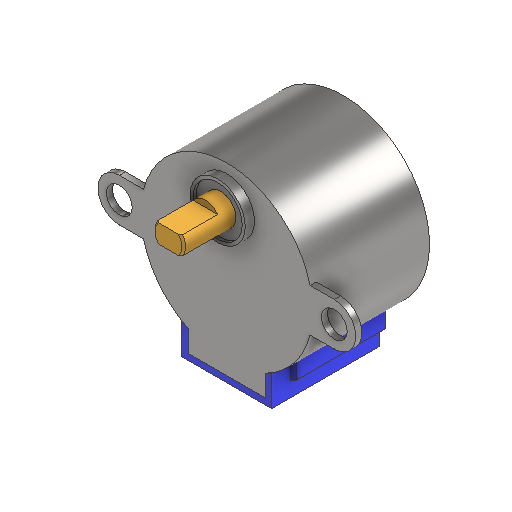
# Autodesk Inventor part: 28BYJ-48 Stepper
Saved by Autodesk Inventor 2023 (Build 270158000, 158)
## iProperties
Created: 2019-05-19
Part Number: 28BYJ-48 Stepper
Material: Generic
Document SubType Name: Modeling
Designer: jotap
Density: 1 g/cm^3
Appearance: Semi-Polished
Author: jotap
Autodesk Inventor part; units mm, degrees
ref_plane "YZ Plane" through (0, 0, 0) normal (1, 0, 0) x (0, 1, 0)
ref_plane "XZ Plane" through (0, 0, 0) normal (0, 1, 0) x (-1, 0, 0)
sketch "Sketch1" plane through (0, 0, 0) normal (0, 0, 1) x (1, 0, 0)
  line L0 (0, 19.6) -> (0, -19.6) construction
  line L1 (-19.6, 0) -> (19.6, 0) construction
  circle A0 centre (0, 0) radius 14
  dimension "d0" = 28
  constraints: 1 centre point, 1 coincident
  measures "d0" diameter of A0
extrude "Extrusion1" add sketch "Sketch1" against normal blind 19
sketch "Sketch2" plane through (0, 0, 0) normal (0, 0, 1) x (1, 0, 0)
  circle A0 centre (0, 0) radius 14 construction
  circle A1 centre (0, 8) radius 4.5
  dimension "d3" = 9
  dimension "d4" = 8
  constraints: 1 centre point
  measures "d3" diameter of A1
  measures "d4" distance of A1.centre A0.centre
extrude "Extrusion2" add sketch "Sketch2" along normal blind 1.5
sketch "Sketch3" plane through (0, 8, 1.5) normal (0, 0, 1) x (1, 0, 0)
  circle A0 centre (0, 0) radius 4.5 construction
  circle A1 centre (0, 0) radius 2.5
  point P0 (0, -8)
  dimension "d7" = 5
  constraints: 1 centre point, 1 coincident
  measures "d7" diameter of A1
extrude "Extrusion3" add sketch "Sketch3" along normal blind 2
sketch "Sketch4" plane through (0, 8, 3.5) normal (0, 0, 1) x (1, 0, 0)
  circle A0 centre (0, 0) radius 2.5 construction
  line L0 (-1.9908, 1.5122) -> (2.0091, 1.4878)
  line L1 (0, 11.6) -> (0, -27.6) construction
  line L2 (-2.6789, 0.0164) -> (3.364, -0.0205) construction
  line L3 (-2.0091, -1.4878) -> (1.9908, -1.5122)
  arc A1 (-1.9908, 1.5122) -> (-2.0091, -1.4878) centre (0, 0) ccw
  arc A2 (1.9908, -1.5122) -> (2.0091, 1.4878) centre (0, 0) ccw
  point P0 (0, -8)
  dimension "d10" = 1.5
  constraints: 6 end point, 4 point on circle, 2 centre point, 2 symmetric about line
  measures "d10" distance from line of L0 A0.centre
extrude "Extrusion4" add sketch "Sketch4" along normal blind 6
chamfer "Chamfer1" distance 0.3 angle 45 2 edges at (2.5, 7.9847, 9.5) (-2.5, 8.0153, 9.5)
sketch "Sketch5" plane through (0, 8, 1.5) normal (0, 0, 1) x (1, 0, 0)
  circle A0 centre (0, 0) radius 4.5 construction
  line L0 (-12.0062, 0) -> (13.0923, 0) construction
  line L1 (0, 11.6) -> (0, -27.6) construction
  circle A1 centre (0, 0) radius 4
  circle A2 centre (0, 0) radius 2.5
  point P0 (0, -8)
  dimension "d16" = 8
  constraints: 2 centre point, 2 coincident, 2 end point, 1 horizontal
  measures "d16" diameter of A1
extrude "Extrusion5" cut sketch "Sketch5" against normal blind 0.5
sketch "Sketch6" plane through (0, 0, 0) normal (0, 0, 1) x (1, 0, 0)
  circle A0 centre (0, 0) radius 14 construction
  arc A1 (-17.5, 3.5) -> (-17.5, -3.5) centre (-17.5, 0) ccw
  line L0 (0, 19.6) -> (0, -19.6) construction
  line L1 (-31.0119, 0) -> (21.502, 0) construction
  circle A2 centre (-17.5, 0) radius 2.1
  line L2 (-17.5, 3.5) -> (-13.5554, 3.5)
  line L3 (-17.5, -3.5) -> (-13.5554, -3.5)
  arc A3 (17.5, -3.5) -> (17.5, 3.5) centre (17.5, 0) ccw
  circle A4 centre (17.5, 0) radius 2.1
  line L4 (17.5, 3.5) -> (13.5554, 3.5)
  line L5 (17.5, -3.5) -> (13.5554, -3.5)
  arc A5 (-13.5554, 3.5) -> (-13.5554, -3.5) centre (0, 0) ccw
  arc A6 (13.5554, -3.5) -> (13.5554, 3.5) centre (0, 0) ccw
  dimension "d19" = 7
  dimension "d20" = 17.5
  dimension "d21" = 4.2
  constraints: 10 point on circle, 8 end point, 6 centre point, 6 symmetric about line, 4 coincident, 2 horizontal, 1 point on line, 2 other
  measures "d19" diameter of A1
  measures "d20" distance of A1.centre A0.centre
  measures "d21" diameter of A2
extrude "Extrusion6" add sketch "Sketch6" against normal blind 1
sketch "Sketch7" plane through (0, 0, 0) normal (0, 0, 1) x (1, 0, 0)
  arc A0 (13.5554, 3.5) -> (-13.5554, 3.5) centre (0, 0) ccw construction
  arc A1 (-13.5554, -3.5) -> (13.5554, -3.5) centre (0, 0) ccw construction
  line L0 (-6.3, -16) -> (6.3, -16)
  line L1 (0, 20) -> (0, -22) construction
  line L2 (-29.4, 0) -> (29.4, 0) construction
  line L3 (-6.3, -16) -> (-6.3, -12.5024)
  line L4 (6.3, -16) -> (6.3, -12.5024)
  arc A2 (-6.3, -12.5024) -> (6.3, -12.5024) centre (0, 0) ccw
  point P0 (0, -16)
  dimension "d24" = 12.6
  dimension "d25" = 16
  constraints: 6 end point, 4 point on circle, 2 vertical, 1 centre point, 1 coincident, 1 horizontal, 1 midpoint, 1 point on line
  measures "d24" distance of L0.start L0.end
  measures "d25" distance from line of L0 A0.centre
extrude "Extrusion7" add sketch "Sketch7" against normal blind 15.5
sketch "Sketch8" plane through (0, 0, 0) normal (0, 0, 1) x (1, 0, 0)
  arc A0 (13.5554, 3.5) -> (-13.5554, 3.5) centre (0, 0) ccw construction
  line L0 (-7.3, -17) -> (7.3, -17)
  line L1 (0, 20.2) -> (0, -23.2) construction
  line L2 (-29.4, 0) -> (29.4, 0) construction
  circle A1 centre (0, 0) radius 14 construction
  line L3 (-6.3, -16) -> (-6.3, -12.5024) construction
  line L4 (6.3, -16) -> (-6.3, -16) construction
  line L5 (-6.3, -16) -> (6.3, -16) construction
  line L6 (-6.31, -16.01) -> (6.31, -16.01)
  arc A2 (-7.3, -11.9578) -> (-6.31, -12.5086) centre (0, 0) ccw
  arc A3 (6.31, -12.5086) -> (7.3, -11.9578) centre (0, 0) ccw
  line L7 (-7.3, -17) -> (-7.3, -11.9578)
  line L8 (-6.31, -16.01) -> (-6.31, -12.5086)
  line L9 (6.31, -16.01) -> (6.31, -12.5086)
  line L10 (7.3, -17) -> (7.3, -11.9578)
  line L11 (6.3, -16) -> (6.3, -12.5024) construction
  point P0 (0, -17)
  point P1 (-6.3, -12.5024)
  point P2 (0, -16.01)
  dimension "d28" = 14.6
  dimension "d29" = 17
  dimension "d34" = 0.01
  dimension "d38" = 14.01
  dimension "d39" = 14.01
  dimension "d42" = 0.01
  dimension "d43" = 0.01
  constraints: 12 end point, 5 point on circle, 4 vertical, 2 centre point, 2 coincident, 2 horizontal, 2 midpoint, 2 point on line
  measures "d28" distance of L0.start L0.end
  measures "d29" distance from line of L0 A0.centre
  measures "d34" distance between parallel lines of L6 L5
  measures "d38" radius of A2
  measures "d39" radius of A3
  measures "d42" distance between parallel lines of L8 L3
  measures "d43" distance between parallel lines of L9 L11
extrude "Extrusion8" add sketch "Sketch8" against normal blind 16.5
sketch "Sketch9" plane through (0, 0, -16.5) normal (0, 0, -1) x (-1, 0, 0)
  line L0 (-7.3, -11.9578) -> (-7.3, -17) projected
  line L1 (-7.3, -17) -> (7.3, -17) projected
  line L2 (7.3, -17) -> (7.3, -11.9578) projected
  circle A0 centre (0, 0) radius 14 construction
  line L3 (7.3, -11.9578) -> (7.3, -17) construction
  line L4 (7.3, -17) -> (-7.3, -17) construction
  line L5 (-7.3, -17) -> (-7.3, -11.9578) construction
  line L6 (0, -23.2) -> (0, 20.2) construction
  line L7 (-29.4, 0) -> (29.4, 0) construction
  arc A1 (-7.3, -11.9578) -> (-6.31, -12.5086) centre (0, 0) ccw construction
  line L8 (7.3, -11.9578) -> (7.3, -17) construction
  arc A2 (-7.3, -11.9578) -> (7.3, -11.9578) centre (0, 0) ccw
  arc A3 (-7.3, -11.9578) -> (-6.31, -12.5086) centre (0, 0) ccw projected
  line L9 (-6.31, -12.5086) -> (-6.31, -16.01) projected
  line L10 (-6.31, -16.01) -> (6.31, -16.01) projected
  line L11 (6.31, -16.01) -> (6.31, -12.5086) projected
  arc A4 (6.31, -12.5086) -> (7.3, -11.9578) centre (0, 0) ccw projected
  constraints: 2 point on circle, 1 centre point, 1 coincident
extrude "Extrusion9" add sketch "Sketch9" along normal blind 1
ref_plane "Work Plane1" through (0, 0, -3) normal (0, 0, 1) x (1, 0, 0)
sketch "Sketch10" plane through (0, 0, -3) normal (0, 0, 1) x (1, 0, 0)
  line L0 (-7.3, -17) -> (-7.3, -11.9578) construction
  arc A0 (-7.3, -11.9578) -> (-6.31, -12.5086) centre (0, 0) ccw construction
  line L1 (-6.31, -12.5086) -> (-6.31, -16.01) construction
  line L2 (-6.31, -16.01) -> (6.31, -16.01) construction
  line L3 (6.31, -16.01) -> (6.31, -12.5086) construction
  arc A1 (6.31, -12.5086) -> (7.3, -11.9578) centre (0, 0) ccw construction
  line L4 (7.3, -11.9578) -> (7.3, -17) construction
  line L5 (7.3, -17) -> (-7.3, -17) construction
  line L6 (-6.3, -16) -> (-6.3, -12.5024) construction
  arc A2 (6.3, -12.5024) -> (-6.3, -12.5024) centre (0, 0) ccw construction
  line L7 (6.3, -12.5024) -> (6.3, -16) construction
  line L8 (6.3, -16) -> (-6.3, -16) construction
  line L9 (-7.3, -17) -> (-7.3, -11.9578) construction
  arc A3 (-7.3, -11.9578) -> (-6.31, -12.5086) centre (0, 0) ccw construction
  line L10 (-6.31, -12.5086) -> (-6.31, -16.01) construction
  line L11 (-6.31, -16.01) -> (6.31, -16.01) construction
  line L12 (6.31, -16.01) -> (6.31, -12.5086) construction
  arc A4 (6.31, -12.5086) -> (7.3, -11.9578) centre (0, 0) ccw construction
  line L13 (7.3, -11.9578) -> (7.3, -17) construction
  line L14 (7.3, -17) -> (-7.3, -17) construction
  line L15 (-6.3, -16) -> (-6.3, -12.5024) construction
  arc A5 (6.3, -12.5024) -> (-6.3, -12.5024) centre (0, 0) ccw construction
  line L16 (6.3, -12.5024) -> (6.3, -16) construction
  line L17 (6.3, -16) -> (-6.3, -16) construction
  line L18 (0, 20.2) -> (0, -23.2) construction
  line L19 (-29.4, 0) -> (29.4, 0) construction
  line L20 (8.3, -14) -> (8.3, -11.2867)
  line L21 (7.3, -11.9578) -> (7.3, -14.5)
  line L22 (7.3, -11.9578) -> (7.3, -17) construction
  line L23 (7.3, -14.5) -> (8.3, -14)
  arc A6 (7.3, -11.9578) -> (8.3, -11.2867) centre (0, 0) ccw
  point P0 (7.3, -11.9578)
  dimension "d45" = 3
  dimension "d46" = 1
  dimension "d47" = 2.5
  dimension "d48" = 14.01
  constraints: 6 end point, 2 point on circle, 2 point on line, 1 centre point, 1 coincident, 1 vertical
  measures "d45" distance from line of L20.start L5
  measures "d46" distance between parallel lines of L4 L20
  measures "d47" distance from line of L21.end L5
  measures "d48" radius of A6
extrude "Extrusion10" add sketch "Sketch10" against normal up to surface (14.5 mm away)
mirror "Mirror1" about plane through (0, 0, 0) normal (1, 0, 0) of "Extrusion10"
sketch "Sketch11" plane through (-7.3, -17, 0) normal (0, -1, 0) x (1, 0, 0)
  line L0 (14.6, -17.5) -> (0, -17.5) construction
  line L1 (0, -17.5) -> (0, 0) construction
  line L2 (0, 0) -> (14.6, 0) construction
  line L3 (14.6, 0) -> (14.6, -17.5) construction
  line L4 (14.6, -17.5) -> (0, -17.5) construction
  line L5 (0, -17.5) -> (0, 0) construction
  line L6 (0, 0) -> (14.6, 0) construction
  line L7 (14.6, 0) -> (14.6, -17.5) construction
  line L8 (14.6, -17.5) -> (0, -17.5) construction
  line L9 (7.3, 15.2) -> (7.3, -24.7) construction
  line L10 (7.3, -24.7) -> (7.3, 15.2) construction
  line L11 (10.8, -15.25) -> (3.8, -15.25) construction
  line L12 (10.8, -14.5) -> (3.8, -14.5)
  line L13 (3.8, -16) -> (10.8, -16)
  arc A0 (10.8, -16) -> (10.8, -14.5) centre (10.8, -15.25) ccw
  arc A1 (3.8, -14.5) -> (3.8, -16) centre (3.8, -15.25) ccw
  point P0 (7.3, 0)
  point P1 (7.3, -15.25)
  dimension "d51" = 7
  dimension "d52" = 1.5
  dimension "d53" = 1.5
  constraints: 8 end point, 4 point on circle, 4 tangent, 2 centre point, 1 horizontal, 1 midpoint, 1 parallel, 1 point on line
  measures "d51" distance of L11.start L11.end
  measures "d52" diameter of A1
  measures "d53" distance between parallel lines of L0 L13
extrude "Extrusion11" cut sketch "Sketch11" against normal blind 10
body "Solid1"
